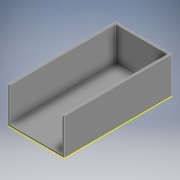
# Autodesk Inventor part: Part1
Saved by Autodesk Inventor 2021 (Build 250183000, 183)
## iProperties
Created: 2023-01-12
Part Number: Part1
Material: Generic
Document SubType Name: Modeling
Designer: boyle
Density: 1 g/cm^3
Appearance: Default
Author: boyle
Autodesk Inventor part; units mm, degrees
ref_plane "YZ Plane" through (0, 0, 0) normal (1, 0, 0) x (0, 1, 0)
ref_plane "XZ Plane" through (0, 0, 0) normal (0, 1, 0) x (-1, 0, 0)
ref_plane "XY Plane" through (0, 0, 0) normal (0, 0, 1) x (1, 0, 0)
sketch "Sketch1" plane through (0, 0, 0) normal (0, 1, 0) x (-1, 0, 0)
  line L0 (0, 0) -> (-107.95, 0)
  line L1 (-107.95, 0) -> (-107.95, 210.82)
  line L2 (-107.95, 210.82) -> (0, 210.82)
  line L3 (0, 210.82) -> (0, 0)
  dimension "d0" = 107.95
  dimension "d1" = 210.82
  constraints: 8 end point, 2 parallel, 1 horizontal, 1 perpendicular
  measures "d0" distance of L1.end L2.end
  measures "d1" distance of L0.end L1.end
extrude "Extrusion1" add sketch "Sketch1" along normal blind 69.85
shell "Shell1" thickness 3.81 removed faces 1 at (71.9667, 69.85, 140.5467)
sketch "Sketch2" plane through (0, 0, 210.82) normal (0, 0, 1) x (1, 0, 0)
  line L0 (0, 0) -> (107.95, 0) projected
  line L1 (107.95, 0) -> (107.95, 69.85) projected
  line L2 (0, 69.85) -> (107.95, 69.85) projected
  line L3 (0, 0) -> (0, 69.85) projected
  point P0 (0, 0)
extrude "Extrusion2" cut sketch "Sketch2" against normal up to surface (3.81 mm away)
sketch "Sketch3" plane through (0, 0, 0) normal (0, -1, 0) x (1, 0, 0)
  line L0 (107.95, 207.01) -> (0, 207.01) projected
  line L1 (0, 0) -> (0, 207.01) projected
  line L2 (107.95, 207.01) -> (107.95, 0) projected
  line L3 (107.95, 207.01) -> (0, 207.01) projected
  line L4 (0, 0) -> (0, 207.01) projected
  line L5 (107.95, 0) -> (0, 0) projected
  line L6 (107.95, 207.01) -> (107.95, 0) projected
  line L7 (107.95, 207.01) -> (107.95, 0) projected
  line L8 (0, 0) -> (0, 207.01) projected
  spline S0 degree 4 poles (107.95, 80.2566) (92.275, 135.0754) (63.1323, -17.4377) (18.2424, 199.5607) (14.8917, 60.7366) (0, 103.505) knots 0 0 0 0 0 0.533015 1 1 1 1 1
  point P0 (82.9333, 90.7317)
  point P1 (54.9148, 82.6505)
  point P2 (27.0432, 108.1624)
  point P3 (14.461, 94.8272)
  point P4 (0, 103.505)
  point P5 (107.95, 80.2566)
  constraints: 1 midpoint, 1 point on line, 6 other
body "Solid1"
